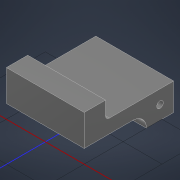
# Autodesk Inventor part: Skirt Mount
Saved by Autodesk Inventor 2022.2 (Build 262287010, 287A)
## iProperties
Created: 2022-03-22
Part Number: Skirt Mount
Material: ABS-Kunststoff
Document SubType Name: Modeling
Designer: sleib
Density: 1.06 g/cm^3
Appearance: Glatt - Schwarz
Author: sleib
Autodesk Inventor part; units mm, degrees
ref_plane "YZ Plane" through (0, 0, 0) normal (1, 0, 0) x (0, 1, 0)
ref_plane "XZ Plane" through (0, 0, 0) normal (0, 1, 0) x (-1, 0, 0)
ref_plane "XY Plane" through (0, 0, 0) normal (0, 0, 1) x (1, 0, 0)
sketch "Skizze1" plane through (0, 0, 0) normal (1, 0, 0) x (0, 1, 0)
  line L0 (0, 0) -> (0, -25)
  line L1 (0, 0) -> (16, 0)
  line L2 (16, 0) -> (16, -39)
  line L3 (9, -46) -> (-7, -46)
  arc A0 (-7, -32) -> (0, -25) centre (-7, -25) ccw
  line L4 (-7, -46) -> (-7, -32)
  arc A1 (9, -46) -> (16, -39) centre (9, -39) ccw
  circle A2 centre (0, -39) radius 7 construction
  circle A3 centre (0, -39) radius 1.7
  arc A4 (9, -11) -> (7, -13) centre (9, -13) ccw
  line L5 (9, -11) -> (16, -11)
  line L6 (7, -13) -> (7, -46)
  dimension "d2" = 14
  dimension "d3" = 16
  dimension "d7" = 14
  dimension "d8" = 3.4
  dimension "d11" = 39
  dimension "d15" = 11
  dimension "d16" = 2
  constraints: 14 end point, 8 tangent, 6 point on circle, 5 centre point, 5 perpendicular, 2 point on line, 1 coincident, 1 equal radius, 1 horizontal, 1 line through centre, 1 vertical, 1 vertical alignment
  measures "d2" distance of L3.end L4.end
  measures "d3" distance of L0.start L1.end
  measures "d7" diameter of A2
  measures "d8" diameter of A3
  measures "d11" distance from line of A2.centre L1
  measures "d15" distance between parallel lines of L5 L1
  measures "d16" radius of A4
extrude "Extrusion1" add sketch "Skizze1" along normal mid plane 40 contours L1 L2 L5 A4 L6 L3 L4 A0 L0
